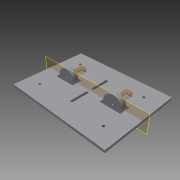
# Autodesk Inventor part: Top
Saved by Autodesk Inventor 2015 (Build 190159000, 159)
## iProperties
Created: 2018-12-21
Part Number: Top
Material: Типовые
Document SubType Name: Modeling
Designer: kostya
Density: 1 g/cm^3
Appearance: По умолчанию
Author: kostya
Autodesk Inventor part; units mm, degrees
ref_plane "YZ Plane" through (0, 0, 0) normal (1, 0, 0) x (0, 1, 0)
ref_plane "XZ Plane" through (0, 0, 0) normal (0, 1, 0) x (-1, 0, 0)
ref_plane "XY Plane" through (0, 0, 0) normal (0, 0, 1) x (1, 0, 0)
sketch "Эскиз1" plane through (0, 0, 0) normal (0, 0, 1) x (1, 0, 0)
  line L0 (-100, -75) -> (100, -75)
  line L1 (100, -75) -> (100, 75)
  line L2 (100, 75) -> (-100, 75)
  line L3 (-100, 75) -> (-100, -75)
  line L4 (-100, -75) -> (100, 75) construction
  line L5 (100, -75) -> (-100, 75) construction
  point P0 (0, 0)
  dimension "d0" = 200
  dimension "d1" = 150
  constraints: 12 end point, 2 midpoint, 2 parallel, 1 horizontal, 1 perpendicular
  measures "d0" distance of L2.end L1.end
  measures "d1" distance of L1.end L0.end
extrude "Выдавливание1" add sketch "Эскиз1" along normal blind 5
sketch "Эскиз2" plane through (0, 0, 5) normal (0, 0, 1) x (1, 0, 0)
  line L0 (100, -75) -> (100, 75) construction
  line L1 (100, 0) -> (-100, 0) construction
  line L2 (-100, 75) -> (-100, -75) construction
  line L3 (100, 75) -> (-100, 75) construction
  line L4 (0, 75) -> (0, -75) construction
  line L5 (-100, -75) -> (100, -75) construction
  line L6 (-100, -10) -> (100, -10) construction
  line L7 (100, -10) -> (100, 10) construction
  line L8 (100, 10) -> (-100, 10) construction
  line L9 (-100, 10) -> (-100, -10) construction
  line L10 (-100, -10) -> (100, 10) construction
  line L11 (100, -10) -> (-100, 10) construction
  line L12 (0, 0) -> (-100, 0) construction
  line L13 (-50, 0) -> (-50, 75) construction
  line L14 (0, 0) -> (100, 0) construction
  line L15 (50, 0) -> (50, 75) construction
  line L16 (-56, 10) -> (-56, 35)
  line L17 (-56, 35) -> (-44, 35)
  line L18 (-44, 35) -> (-44, 10)
  line L19 (-56, 10) -> (-44, 10)
  line L20 (56, 10) -> (56, 35)
  line L21 (56, 35) -> (44, 35)
  line L22 (44, 35) -> (44, 10)
  line L23 (56, 10) -> (44, 10)
  line L24 (-70, -10) -> (-30, -10)
  line L25 (-30, -10) -> (-30, 10)
  line L26 (-30, 10) -> (-70, 10)
  line L27 (-70, 10) -> (-70, -10)
  line L28 (-70, -10) -> (-30, 10) construction
  line L29 (-30, -10) -> (-70, 10) construction
  line L30 (70, -10) -> (30, -10)
  line L31 (30, -10) -> (30, 10)
  line L32 (30, 10) -> (70, 10)
  line L33 (70, 10) -> (70, -10)
  dimension "d4" = 20
  dimension "d7" = 25
  dimension "d8" = 40
  constraints: 60 end point, 10 midpoint, 8 symmetric about line, 7 perpendicular, 6 point on line, 4 parallel, 2 collinear, 2 horizontal, 1 vertical
  measures "d4" distance of L7.end L6.end
  measures "d7" distance of L16.start L16.end
  measures "d8" distance of L26.end L25.end
extrude "Выдавливание2" cut sketch "Эскиз2" against normal blind 2 contours L16 L17 L18 L19 | L23 L22 L21 L20
extrude "Выдавливание3" cut sketch "Эскиз2" against normal blind 5 contours L19 L26 L25 L24 L27 | L32 L33 L30 L31 L23
sketch "Эскиз3" plane through (0, 0, 3) normal (0, 0, 1) x (1, 0, 0)
  line L0 (-56, 10) -> (-56, 35) projected
  line L1 (-44, 10) -> (-56, 10) projected
  line L2 (-44, 35) -> (-44, 10) projected
  line L3 (-56, 35) -> (-44, 35) projected
  line L4 (-44, 35) -> (-44, 10) projected
  point P0 (0, 0)
surface extrude "ВыдавПврх1" sketch "Эскиз3" along normal blind 10 shown yes curves L4 L1 L0 L3
boundary_patch "Участок поверхности1"
sketch "Эскиз4" plane through (-56, 10, 3) normal (0, -1, 0) x (1, 0, 0)
  line L0 (0, 10) -> (12, 10) construction
  line L1 (6, 10) -> (6, 0) construction
  line L2 (12, 0) -> (0, 0) construction
  line L3 (0, 0) -> (0, 10) construction
  line L4 (0, 5) -> (12, 5) construction
  line L5 (12, 0) -> (12, 10) construction
  arc A0 (7.118, 4) -> (4.882, 4) centre (6, 5) ccw
  line L6 (6, 3.5) -> (6, 4) construction
  line L7 (6, 4) -> (7.118, 4)
  line L8 (6, 4) -> (4.882, 4)
  point P0 (56, -3)
  dimension "d17" = 3
  dimension "d18" = 0.5
  constraints: 10 end point, 5 midpoint, 2 point on circle, 2 point on line, 1 centre point, 1 horizontal, 1 perpendicular
  measures "d17" diameter of A0
  measures "d18" distance of L6.start L6.end
surface extrude "ВыдавПврх2" sketch "Эскиз4" along normal blind 10 shown yes curves L7 A0 L8
boundary_patch "Участок поверхности2"
mirror "Зеркальное отражение1" about plane through (0, 0, 0) normal (1, 0, 0) of "Участок поверхности1", "ВыдавПврх1", "ВыдавПврх2"
ref_plane "РабПлоскость1" through (-70, 0, 5) normal (0, -1, 0) x (1, 0, 0)
sketch "Эскиз5" plane through (-70, 0, 5) normal (0, -1, 0) x (1, 0, 0)
  arc A0 (21.118, 2) -> (18.882, 2) centre (20, 3) ccw projected
  line L0 (18.882, 2) -> (21.118, 2) projected
  circle A1 centre (20, 3) radius 17.5
  point P0 (70, -5)
  dimension "d23" = 35
  constraints: 1 centre point, 1 coincident
  measures "d23" diameter of A1
extrude "Выдавливание4" add sketch "Эскиз5" along normal mid plane 10
mirror "Зеркальное отражение2" about plane through (0, 0, 0) normal (1, 0, 0) of "Выдавливание4"
sketch "Эскиз6" plane through (0, 0, 5) normal (0, 0, 1) x (1, 0, 0)
  line L0 (-100, -75) -> (100, -75) projected
  line L1 (100, -75) -> (100, 75) projected
  line L2 (100, 75) -> (-100, 75) projected
  line L3 (-100, 75) -> (-100, -75) projected
  line L4 (-44, 10) -> (-30, 10) projected
  line L5 (-30, 10) -> (-30, -10) projected
  line L6 (-30, -10) -> (-70, -10) projected
  line L7 (-70, -10) -> (-70, 10) projected
  line L8 (-70, 10) -> (-56, 10) projected
  line L9 (-56, 10) -> (-56, 35) projected
  line L10 (-56, 35) -> (-44, 35) projected
  line L11 (-44, 35) -> (-44, 10) projected
  line L12 (30, 10) -> (44, 10) projected
  line L13 (44, 10) -> (44, 35) projected
  line L14 (44, 35) -> (56, 35) projected
  line L15 (56, 35) -> (56, 10) projected
  line L16 (56, 10) -> (70, 10) projected
  line L17 (70, 10) -> (70, -10) projected
  line L18 (70, -10) -> (30, -10) projected
  line L19 (30, -10) -> (30, 10) projected
  line L20 (100, -75) -> (70, -75)
  line L21 (70, -75) -> (70, -45) construction
  line L22 (70, -45) -> (100, -45) construction
  line L23 (100, -45) -> (100, -75)
  circle A0 centre (70, -45) radius 2.5
  line L24 (-100, 0) -> (100, 0) construction
  line L25 (100, 75) -> (-100, 75) construction
  line L26 (0, 75) -> (0, -75) construction
  circle A1 centre (-70, -45) radius 2.5
  circle A2 centre (70, 45) radius 2.5
  circle A3 centre (-70, 45) radius 2.5
  point P0 (0, 0)
  dimension "d26" = 30
  dimension "d27" = 30
  dimension "d28" = 5
  constraints: 12 end point, 5 symmetric about line, 4 centre point, 4 midpoint, 3 coincident, 2 parallel, 1 horizontal, 1 perpendicular, 3 other
  measures "d26" distance of L21.end L22.end
  measures "d27" distance of L20.end L21.end
  measures "d28" diameter of A0
extrude "Выдавливание5" cut sketch "Эскиз6" against normal blind 10 contours A0 | A1 | A2 | A3
sketch "Эскиз7" plane through (0, 0, 5) normal (0, 0, 1) x (1, 0, 0)
  circle A0 centre (-70, 45) radius 2.5 projected
  circle A1 centre (70, -45) radius 2.5 projected
  circle A2 centre (-70, -45) radius 2.5 projected
  circle A3 centre (70, 45) radius 2.5 projected
  line L0 (-100, -75) -> (100, -75) projected
  line L1 (100, -75) -> (100, 75) projected
  line L2 (100, 75) -> (-100, 75) projected
  line L3 (-100, 75) -> (-100, -75) projected
  line L4 (-44, 10) -> (-30, 10) projected
  line L5 (-30, 10) -> (-30, -10) projected
  line L6 (-30, -10) -> (-70, -10) projected
  line L7 (-70, -10) -> (-70, 10) projected
  line L8 (-70, 10) -> (-56, 10) projected
  line L9 (-56, 10) -> (-56, 35) projected
  line L10 (-56, 35) -> (-44, 35) projected
  line L11 (-44, 35) -> (-44, 10) projected
  line L12 (30, 10) -> (44, 10) projected
  line L13 (44, 10) -> (44, 35) projected
  line L14 (44, 35) -> (56, 35) projected
  line L15 (56, 35) -> (56, 10) projected
  line L16 (56, 10) -> (70, 10) projected
  line L17 (70, 10) -> (70, -10) projected
  line L18 (70, -10) -> (30, -10) projected
  line L19 (30, -10) -> (30, 10) projected
  line L20 (100, 75) -> (-100, 75) construction
  line L21 (-30, 10) -> (30, 10) construction
  line L22 (30, 10) -> (30, 75) construction
  line L23 (30, 75) -> (-30, 75) construction
  line L24 (-30, 75) -> (-30, 10) construction
  line L25 (-100, -75) -> (100, -75) construction
  line L26 (-30, -10) -> (30, -10) construction
  line L27 (30, -10) -> (30, -75) construction
  line L28 (30, -75) -> (-30, -75) construction
  line L29 (-30, -75) -> (-30, -10) construction
  line L30 (100, -75) -> (100, 75) construction
  line L31 (100, -7.5) -> (100, 7.5) construction
  line L32 (100, 7.5) -> (-100, 7.5) construction
  line L33 (-100, 7.5) -> (-100, -7.5) construction
  line L34 (-100, -7.5) -> (100, 7.5) construction
  line L35 (100, -7.5) -> (-100, 7.5) construction
  line L36 (-100, -7.5) -> (-2.5, -7.5) construction
  line L37 (2.5, -7.5) -> (100, -7.5) construction
  line L38 (-100, 75) -> (-100, -75) construction
  line L39 (-100, 0) -> (100, 0) construction
  arc A4 (-2.5, 7.5) -> (2.5, 7.5) centre (0, 7.5) ccw
  line L40 (2.5, 7.5) -> (2.5, 38.1)
  line L41 (-2.5, 38.1) -> (-2.5, 7.5)
  arc A5 (2.5, 38.1) -> (-2.5, 38.1) centre (0, 38.1) ccw
  line L42 (-2.5, 38.1) -> (-2.5, 7.5)
  line L43 (2.5, 7.5) -> (2.5, 38.1)
  line L44 (-2.5, -38.1) -> (-2.5, -7.5)
  line L45 (2.5, -7.5) -> (2.5, -38.1)
  arc A6 (-2.5, -38.1) -> (2.5, -38.1) centre (0, -38.1) ccw
  arc A7 (2.5, -7.5) -> (-2.5, -7.5) centre (0, -7.5) ccw
  point P0 (0, 0)
  dimension "d31" = 15
  constraints: 44 end point, 8 parallel, 8 point on circle, 6 symmetric about line, 4 centre point, 4 horizontal, 4 midpoint, 4 perpendicular, 4 point on line, 1 collinear, 1 other
  measures "d31" distance of L31.end L31.start
extrude "Выдавливание7" cut sketch "Эскиз7" against normal blind 10 contours L41 A5 L40 A4 | L44 A7 L45 A6
body "SRF1"
body "SRF2"
body "SRF3"
body "SRF4"
body "SRF5"
body "SRF6"
body "SRF7"
